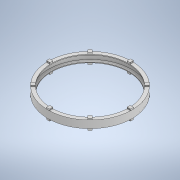
# Autodesk Inventor part: Ring
Saved by Autodesk Inventor 2022 (Build 260153000, 153)
## iProperties
Created: 2021-12-15
Part Number: Ring
Material: Generic
Document SubType Name: Sheet Metal
Designer: lcroo
Density: 1 g/cm^3
Sheet Metal Rule: Default_mm
Appearance: Default
Author: lcroo
Autodesk Inventor part; units mm, degrees
sketch "Sketch1" plane through (0, 0, 0) normal (0, 1, 0) x (-1, 0, 0)
  circle A0 centre (0, 0) radius 140
  circle A1 centre (0, 0) radius 128.5
  dimension "d0" = 280
  dimension "d1" = 257
  constraints: 2 centre point, 2 coincident
  measures "d0" diameter of A0
  measures "d1" diameter of A1
extrude "Extrusion1" add sketch "Sketch1" along normal blind 25
ref_plane "Work Plane1" through (0, 12.5, 0) normal (0, 1, 0) x (1, 0, 0)
ref_plane "Work Plane3" through (0, 12.5, 0) normal (0, 1, 0) x (1, 0, 0)
sketch "Sketch8" plane through (0, 12.5, 0) normal (0, 1, 0) x (1, 0, 0)
  circle A0 centre (0, 0) radius 139
  circle A1 centre (0, 0) radius 128.5
  dimension "d21" = 278
  dimension "d22" = 257
  constraints: 2 centre point, 2 coincident
  measures "d21" diameter of A0
  measures "d22" diameter of A1
extrude "Extrusion5" cut sketch "Sketch8" along normal mid plane 20
sketch "Sketch9" plane through (0, 25, 0) normal (0, 1, 0) x (1, 0, 0)
  circle A0 centre (0, 0) radius 140 projected
  line L0 (-140, 0) -> (-128.5, 0)
  line L1 (-128.5, 0) -> (-128.5, 5)
  line L2 (-128.5, 5) -> (-140, 5)
  line L3 (-140, 5) -> (-140, 0)
  dimension "d25" = 5
  constraints: 8 end point, 2 parallel, 1 horizontal, 1 horizontal alignment, 1 perpendicular, 1 other
  measures "d25" distance of L1.end L0.end
extrude "Extrusion6" add sketch "Sketch9" along normal blind 5 contours L3 L2 A0 | A0 L2 L1 L0 picked at (-132.3201, 2.7779)
sketch "Sketch10" plane through (0, 25, 0) normal (0, 1, 0) x (1, 0, 0)
  line L0 (0, 0) -> (0, 140)
  circle A0 centre (0, 0) radius 140 projected
  line L1 (0, 0) -> (0, -140)
  line L2 (-140, 0) -> (140, 0)
  line L3 (85.4982, 110.8605) -> (221.3583, 110.8605) construction
  line L4 (0, 0) -> (98.9949, -98.9949)
  line L5 (0, 0) -> (140, 0) construction
  line L6 (140, 0) -> (-140, 0)
  line L7 (0, 0) -> (-98.9949, -98.9949)
  line L8 (0, 0) -> (98.9949, 98.9949)
  line L9 (0, 0) -> (-98.9949, 98.9949)
  line L10 (0, 0) -> (-129.3431, 53.5757)
  dimension "d29" = 45
  dimension "d30" = 22.5
  dimension "d31" = 22.5
  constraints: 22 end point, 5 symmetric about line, 2 horizontal, 1 equal length, 1 perpendicular, 1 point on line, 1 vertical, 8 other
  measures "d29" angle of L4 L5
  measures "d30" angle of L10 L9
  measures "d31" angle of L2 L10
sketch "Sketch11" plane through (-140, 25, 0) normal (0, 0, 1) x (1, 0, 0)
  circle A0 centre (3, 2.5) radius 1
  circle A1 centre (8.5, 2.5) radius 1
  line L0 (0, 0) -> (0, 5) projected
  line L1 (11.5, 0) -> (11.5, 5) projected
  line L2 (0, 5) -> (11.5, 5) projected
  point P0 (140, -25)
  dimension "d32" = 2
  dimension "d33" = 2
  dimension "d34" = 3
  dimension "d36" = 3
  dimension "d37" = 2.5
  dimension "d38" = 2.5
  constraints: 2 centre point
  measures "d32" diameter of A0
  measures "d33" diameter of A1
  measures "d34" distance from line of L0 A0.centre
  measures "d36" distance from line of L1 A1.centre
  measures "d37" distance from line of L2 A0.centre
  measures "d38" distance from line of L2 A1.centre
extrude "Extrusion7" cut sketch "Sketch11" against normal blind 5
ref_plane "Work Plane4" through (0, 25, 0) normal (0.3826834, 0, -0.9238795) x (-0.9238795, 0, -0.3826834)
mirror "Mirror1" about plane through (0, 25, 0) normal (0.3826834, 0, -0.9238795) of "Extrusion6", "Extrusion7"
ref_plane "Work Plane5" through (0, 25, 0) normal (0.7071068, 0, -0.7071068) x (-0.7071068, 0, -0.7071068)
ref_plane "Work Plane6" through (0, 25, 0) normal (1, 0, 0) x (0, 0, -1)
ref_plane "Work Plane7" through (0, 25, 0) normal (0.7071068, 0, 0.7071068) x (0.7071068, 0, -0.7071068)
ref_plane "Work Plane8" through (0, 25, 0) normal (0, 0, 1) x (1, 0, 0)
pattern_circular "Circular Pattern1" count 8 over 360 about axis through (0, -10, 0) along (0, 1, 0) of "Extrusion7", "Extrusion6", "Mirror1"
ref_plane "Work Plane9" through (0, 12.5, 0) normal (0, 1, 0) x (1, 0, 0)
mirror "Mirror2" about plane through (0, 12.5, 0) normal (0, 1, 0) of "Extrusion7", "Extrusion6", "Mirror1", "Circular Pattern1"
sketch "Sketch12" plane through (-94.3988, 30, -87.3277) normal (0, 1, 0) x (0.7071068, 0, -0.7071068)
  line L0 (10, 11.5) -> (0, 11.5) projected
  line L1 (5, 11.5) -> (5, 0)
  line L2 (10, 0) -> (0, 0) projected
  point P0 (5, -128.5)
  constraints: 2 end point, 2 midpoint
sketch "Sketch13" plane through (-102.5305, -5, -95.4594) normal (0, -1, 0) x (0.7071068, 0, -0.7071068)
  arc A0 (5, 0) -> (10, 0.0893) centre (5, 140) ccw projected
  line L0 (5, 11.5) -> (10, 11.5) projected
  line L1 (5, 0) -> (5, 11.5)
  point P0 (5, 140)
  constraints: 2 end point, 1 point on circle, 1 vertical
equation "\"BendRadius\" = Thickness"
equation "\"BendReliefWidth\" = Thickness"
equation "\"BendReliefDepth\" = 0.5 * Thickness"
equation "\"CornerReliefSize\" = 4 * Thickness"
equation "\"MinimumRemnant\" = 2 * Thickness"
equation "\"TransitionRadius\" = BendRadius"
equation "\"JacobiRadiusSize\" = BendRadius"
equation "\"GapSize\" = Thickness"
equation "\"Thickness\" = 0.5"
body "Solid1"
